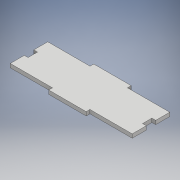
# Autodesk Inventor part: F4
Saved by Autodesk Inventor 2018 (Build 220112000, 112)
## iProperties
Created: 2018-03-06
Part Number: F4
Material: Generic
Document SubType Name: Modeling
Designer: isai
Density: 1 g/cm^3
Appearance: Default
Author: isai
Autodesk Inventor part; units mm, degrees
ref_plane "YZ Plane" through (0, 0, 0) normal (1, 0, 0) x (0, 1, 0)
ref_plane "XZ Plane" through (0, 0, 0) normal (0, 1, 0) x (-1, 0, 0)
sketch "Sketch1" plane through (0, 0, 0) normal (0, 0, 1) x (1, 0, 0)
  line L0 (-101, -254.2) -> (-101, -258.2)
  line L1 (-101, -258.2) -> (-56, -258.2)
  line L2 (-56, -258.2) -> (-56, -254.2)
  line L3 (-56, -254.2) -> (-16, -254.2)
  line L4 (-16, -254.2) -> (-16, -258.2)
  line L5 (-16, -258.2) -> (29, -258.2)
  line L6 (29, -258.2) -> (29, -254.2)
  line L7 (-101, -258.2) -> (-101, -298.2)
  line L8 (29, -258.2) -> (29, -298.2)
  line L9 (29, -278.2) -> (70.7342, -278.2)
  line L10 (-56, -298.2) -> (-56, -302.2)
  line L11 (-56, -302.2) -> (-16, -302.2)
  line L12 (-16, -302.2) -> (-16, -298.2)
  line L13 (-101, -298.2) -> (-56, -298.2)
  line L14 (-16, -298.2) -> (29, -298.2)
  point P0 (0, 0)
  dimension "d0" = 40
  dimension "d1" = 40
  dimension "d2" = 130
  constraints: 30 end point, 4 symmetric about line, 2 perpendicular, 2 point on line, 2 vertical, 1 horizontal, 1 midpoint
  measures "d0" distance of L0.end L7.end
  measures "d1" distance of L2.end L3.end
  measures "d2" distance of L7.end L8.end
extrude "Extrusion1" add sketch "Sketch1" along normal blind 4
sketch "Sketch2" plane through (0, 0, 4) normal (0, 0, 1) x (1, 0, 0)
  line L0 (-56, -258.2) -> (-101, -258.2) projected
  line L1 (-101, -258.2) -> (-101, -298.2) projected
  line L2 (-101, -298.2) -> (-56, -298.2) projected
  line L3 (-56, -298.2) -> (-56, -302.2) projected
  line L4 (-56, -302.2) -> (-16, -302.2) projected
  line L5 (-16, -302.2) -> (-16, -298.2) projected
  line L6 (-16, -298.2) -> (29, -298.2) projected
  line L7 (29, -298.2) -> (29, -258.2) projected
  line L8 (29, -258.2) -> (-16, -258.2) projected
  line L9 (-16, -258.2) -> (-16, -254.2) projected
  line L10 (-16, -254.2) -> (-56, -254.2) projected
  line L11 (-56, -254.2) -> (-56, -258.2) projected
  line L12 (25, -273.2) -> (29, -273.2)
  line L13 (29, -273.2) -> (29, -283.2)
  line L14 (29, -283.2) -> (25, -283.2)
  line L15 (25, -283.2) -> (25, -273.2)
  point P0 (0, 0)
  point P1 (29, -278.2)
  dimension "d5" = 4
  dimension "d6" = 10
  constraints: 8 end point, 2 midpoint, 2 parallel, 1 horizontal, 1 perpendicular
  measures "d5" distance of L13.end L14.end
  measures "d6" distance of L12.end L13.end
extrude "Extrusion2" cut sketch "Sketch2" against normal blind 4 contours L7 L14 L15 L12
ref_plane "Work Plane1" through (-36, -258.2, 4) normal (1, 0, 0) x (0, 0, -1)
mirror "Mirror1" about plane through (-36, -258.2, 4) normal (1, 0, 0) of "Extrusion2"
body "Solid1"
